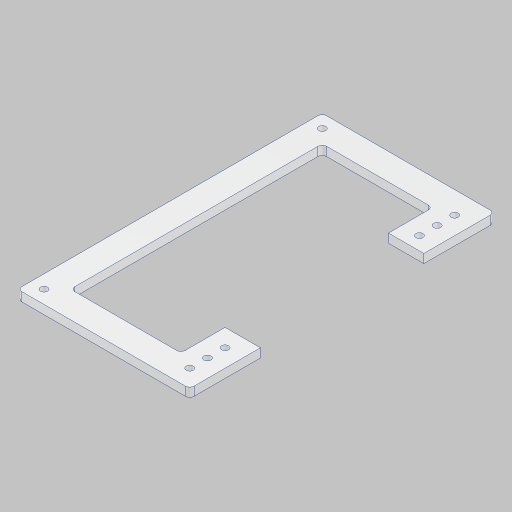
# Autodesk Inventor part: DB1-009
Saved by Autodesk Inventor 2023.5 (Build 275446000, 446)
## iProperties
Created: 2025-01-31
Part Number: DB1-009
Material: Aluminum 6061
Document SubType Name: Modeling
Designer: 27karwoodwills
Density: 2.7 g/cm^3
Appearance: Aluminum - Flat
Author: 27karwoodwills
Autodesk Inventor part; units mm, degrees
ref_plane "YZ Plane" through (0, 0, 0) normal (1, 0, 0) x (0, 1, 0)
ref_plane "XZ Plane" through (0, 0, 0) normal (0, 1, 0) x (-1, 0, 0)
ref_plane "XY Plane" through (0, 0, 0) normal (0, 0, 1) x (1, 0, 0)
sketch "Sketch1" plane through (0, 0, 0) normal (0, 1, 0) x (-1, 0, 0)
  line L0 (0, 0) -> (79.375, 0)
  line L1 (79.375, 0) -> (79.375, 19.05) construction
  line L2 (79.375, 19.05) -> (0, 19.05)
  line L3 (0, 19.05) -> (0, 0) construction
  line L4 (79.375, 19.05) -> (98.425, 19.05)
  line L5 (98.425, 19.05) -> (98.425, -200.025)
  line L6 (98.425, -200.025) -> (79.375, -200.025)
  line L7 (79.375, -200.025) -> (79.375, 19.05)
  line L8 (79.375, -200.025) -> (0, -200.025)
  line L9 (0, -200.025) -> (0, -180.975) construction
  line L10 (0, -180.975) -> (79.375, -180.975)
  line L11 (79.375, -180.975) -> (79.375, -200.025) construction
  line L12 (0, 0) -> (-25.4, 0) construction
  line L13 (-25.4, 0) -> (-25.4, 19.05)
  line L14 (-25.4, 19.05) -> (0, 19.05)
  line L15 (0, 19.05) -> (0, 0)
  line L16 (0, -180.975) -> (-25.4, -180.975) construction
  line L17 (-25.4, -180.975) -> (-25.4, -200.025)
  line L18 (-25.4, -200.025) -> (0, -200.025)
  line L19 (0, -200.025) -> (0, -180.975) construction
  circle A0 centre (-12.7, 6.35) radius 2.54 construction
  circle A1 centre (-12.7, -187.325) radius 2.54 construction
  circle A2 centre (88.9, -190.5) radius 2.54 construction
  circle A3 centre (88.9, 9.525) radius 2.54 construction
  line L20 (0, -180.975) -> (-25.4, -180.975) construction
  line L21 (-25.4, -180.975) -> (-25.4, -149.225)
  line L22 (-25.4, -149.225) -> (0, -149.225)
  line L23 (0, -149.225) -> (0, -180.975)
  line L24 (0, -180.975) -> (-25.4, -149.225) construction
  line L25 (-25.4, -180.975) -> (0, -149.225) construction
  line L26 (0, -31.75) -> (-25.4, -31.75)
  line L27 (-25.4, -31.75) -> (-25.4, 0)
  line L28 (-25.4, 0) -> (0, 0) construction
  line L29 (0, 0) -> (0, -31.75)
  line L30 (0, -31.75) -> (-25.4, 0) construction
  line L31 (-25.4, -31.75) -> (0, 0) construction
  point P0 (79.375, 0)
  point P1 (79.375, -180.975)
  point P2 (0, -200.025)
  point P3 (79.375, -190.5)
  point P4 (0, -200.025)
  point P5 (-12.7, -165.1)
  point P6 (-12.7, -15.875)
  dimension "d0" = 79.375
  dimension "d1" = 19.05
  dimension "d3" = 19.05
  dimension "d4" = 79.375
  dimension "d5" = 19.05
  dimension "d8" = 180.975
  dimension "d9" = 25.4
  dimension "d10" = 19.05
  dimension "d11" = 25.4
  dimension "d12" = 19.05
  dimension "d17" = 5.08
  dimension "d18" = 6.35
  dimension "d20" = 5.08
  dimension "d21" = 12.7
  dimension "d23" = 12.7
  dimension "d38" = 5.08
  dimension "d39" = 9.525
  dimension "d40" = 9.525
  dimension "d41" = 5.08
  dimension "d42" = 9.525
  dimension "d43" = 9.525
  dimension "d52" = 12.7
  dimension "d53" = 25.4
  dimension "d54" = 50.8
  dimension "d55" = 50.8
  dimension "d56" = 25.4
  constraints: 64 end point, 14 parallel, 7 horizontal, 7 perpendicular, 5 midpoint, 4 centre point, 4 coincident
  measures "d0" distance of L2.end L1.end
  measures "d1" distance of L1.end L0.end
  measures "d3" distance of L5.end L6.end
  measures "d4" distance of L9.end L10.end
  measures "d5" distance of L8.end L9.end
  measures "d8" distance between parallel lines of L10 L0
  measures "d9" distance of L13.end L14.end
  measures "d10" distance of L12.end L13.end
  measures "d11" distance of L18.end L17.end
  measures "d12" distance of L17.end L16.end
  measures "d17" diameter of A0
  measures "d18" distance from line of A0.centre L12
  measures "d20" diameter of A1
  measures "d21" distance from line of L18 A1.centre
  measures "d23" distance from line of point (-12.7, 6.35) L13
  measures "d38" diameter of A2
  measures "d39" distance from line of A2.centre L6
  measures "d40" distance of A2.centre point (79.375, -190.5)
  measures "d41" diameter of A3
  measures "d42" distance from line of L4 A3.centre
  measures "d43" distance from line of L5 A3.centre
  measures "d52" distance from line of A1.centre L17
  measures "d53" distance of L21.end L22.end
  measures "d54" distance between parallel lines of L22 L18
  measures "d55" distance between parallel lines of L14 L26
  measures "d56" distance of L26.start L26.end
extrude "Extrusion1" add sketch "Sketch1" along normal blind 6.35
hole "Hole3" at (-88.9, 0, -190.5) at (-88.9, 0, 9.525) direction (0, 1, 0) diameter 5.1054 end through all clearance for "Flat Head Machine Screw (82)" size "#10" standard "Ansi Unified Screw Threads"
fillet "Fillet1" radius 3.175 8 edges at (-98.425, 3.175, -200.025) (25.4, 3.175, -200.025) (-79.375, 3.175, -180.975) (-79.375, 3.175, 0) (-98.425, 3.175, 19.05) (25.4, 3.175, 19.05) (0, 3.175, 0) (0, 3.175, -180.975)
sketch "Sketch3" plane through (0, 6.35, 0) normal (0, 1, 0) x (1, 0, 0)
  line L0 (-95.25, -19.05) -> (22.225, -19.05) construction
  line L1 (25.4, -15.875) -> (25.4, 31.75) construction
  point P0 (0, 0)
  point P1 (12.7, -6.35)
  point P2 (12.7, 6.35)
  point P3 (12.7, 19.05)
  point P4 (12.7, 31.75)
  point P5 (12.7, 44.45)
  point P6 (12.7, 57.15)
  point P7 (12.7, 69.85)
  point P8 (12.7, 82.55)
  point P9 (12.7, 95.25)
  point P10 (12.7, 107.95)
  point P11 (12.7, 120.65)
  point P12 (12.7, 133.35)
  point P13 (12.7, 146.05)
  point P14 (12.7, 158.75)
  point P15 (12.7, 171.45)
  point P16 (12.7, 184.15)
  dimension "d57" = 12.7
  dimension "d58" = 12.7
  dimension "d61" = 12.7
  constraints: 1 vertical, 15 other
  measures "d57" distance from line of L0 point (12.7, -6.35)
  measures "d58" distance from line of L1 point (12.7, -6.35)
  measures "d61" distance of point (12.7, -6.35) point (12.7, 6.35)
hole "Hole4" at (12.7, 6.35, 6.35) at (12.7, 6.35, -6.35) at (12.7, 6.35, -19.05) at (12.7, 6.35, -44.45) at (12.7, 6.35, -57.15) at (12.7, 6.35, -69.85) at (12.7, 6.35, -82.55) at (12.7, 6.35, -95.25) at (12.7, 6.35, -107.95) at (12.7, 6.35, -120.65) at (12.7, 6.35, -133.35) at (12.7, 6.35, -146.05) at (12.7, 6.35, -158.75) at (12.7, 6.35, -171.45) at (12.7, 6.35, -184.15) direction (0, -1, 0) diameter 5.1054 end through all clearance for "Flat Head Machine Screw (82)" size "#10" standard "Ansi Unified Screw Threads"
equation "\"d4\" = d0"
body "Solid1"
